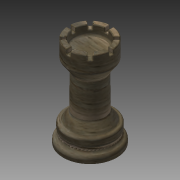
# Autodesk Inventor part: Castle
Saved by Autodesk Inventor 2015 SP1 (Build 190203100, 203)
## iProperties
Created: 2015-06-07
Part Number: Castle
Material: Generic
Document SubType Name: Modeling
Designer: Nathan
Density: 1 g/cm^3
Appearance: Driftwood
Author: Nathan
Autodesk Inventor part; units mm, degrees
ref_plane "YZ Plane" through (0, 0, 0) normal (1, 0, 0) x (0, 1, 0)
ref_plane "XZ Plane" through (0, 0, 0) normal (0, 1, 0) x (-1, 0, 0)
ref_plane "XY Plane" through (0, 0, 0) normal (0, 0, 1) x (1, 0, 0)
sketch "Sketch1" plane through (0, 0, 0) normal (0, 0, 1) x (1, 0, 0)
  line L0 (0, 47) -> (0, 0)
  line L1 (0, 0) -> (14.846, 0)
  arc A0 (12.9584, 6.4952) -> (13.7958, 3.4613) centre (14.831, 5.3796) ccw
  line L2 (13.2402, 9.7167) -> (13.2402, 7.5188)
  line L3 (14.846, 1.7013) -> (14.846, 0)
  arc A1 (12.9584, 6.4952) -> (13.2402, 7.5188) centre (11.2402, 7.5188) ccw
  arc A2 (14.846, 1.7013) -> (13.7958, 3.4613) centre (12.846, 1.7013) ccw
  arc A3 (13.2402, 9.7167) -> (12.1426, 10.7119) centre (12.2402, 9.7167) ccw
  arc A4 (11.2263, 11.133) -> (12.1426, 10.7119) centre (12.045, 11.7072) ccw
  line L4 (0, 0) -> (0, 50)
  line L5 (0, 50) -> (12.0578, 50)
  line L6 (12.0578, 50) -> (12.0578, 41.4087)
  line L7 (11.6943, 40.259) -> (8.3296, 35.4699)
  line L8 (7.9662, 34.2984) -> (8.1644, 16.1086)
  line L9 (8.5268, 14.982) -> (11.2263, 11.133)
  arc A5 (11.6943, 40.259) -> (12.0578, 41.4087) centre (10.0578, 41.4087) ccw
  arc A6 (8.3296, 35.4699) -> (7.9662, 34.2984) centre (9.9661, 34.3202) ccw
  arc A7 (8.1644, 16.1086) -> (8.5268, 14.982) centre (10.1642, 16.1304) ccw
  point P0 (14.846, 3.1999)
  point P1 (13.2402, 6.8697)
  point P2 (12.2402, 10.7167)
  point P3 (7.9592, 34.9427)
  point P4 (8.1711, 15.4891)
  dimension "d11" = 2
  dimension "d13" = 1
  dimension "d14" = 1
  dimension "d17" = 50
  dimension "d20" = 2
  constraints: 20 end point, 19 point on circle, 13 tangent, 8 centre point, 7 point on line, 3 equal radius, 2 horizontal, 2 vertical, 1 perpendicular
  measures "d11" radius of A1
  measures "d13" radius of A3
  measures "d14" radius of A4
  measures "d17" distance of L0.end L4.end
  measures "d20" radius of A5
revolve "Revolution1" add sketch "Sketch1" angle 360 about axis through (0, 47, 0) along (0, -1, 0)
sketch "Sketch2" plane through (0, 50, 0) normal (0, 1, 0) x (1, 0, 0)
  circle A0 centre (0, 0) radius 9
  dimension "d21" = 18
  constraints: 1 centre point, 1 coincident
  measures "d21" diameter of A0
extrude "Extrusion1" cut sketch "Sketch2" against normal blind 5
sketch "Sketch3" plane through (0, 50, 0) normal (0, 1, 0) x (1, 0, 0)
  line L0 (-1, -2.4142) -> (-12.1516, -13.5658)
  line L1 (-1, -18.185) -> (-1, -2.4142)
  line L2 (-2.4142, -1) -> (-18.185, -1)
  line L3 (-13.5658, -12.1516) -> (-2.4142, -1)
  line L4 (-2.4142, 1) -> (-13.5658, 12.1516)
  line L5 (-18.185, 1) -> (-2.4142, 1)
  line L6 (-1, 2.4142) -> (-1, 18.185)
  line L7 (-12.1516, 13.5658) -> (-1, 2.4142)
  line L8 (1, 2.4142) -> (12.1516, 13.5658)
  line L9 (1, 18.185) -> (1, 2.4142)
  line L10 (2.4142, 1) -> (18.185, 1)
  line L11 (13.5658, 12.1516) -> (2.4142, 1)
  line L12 (2.4142, -1) -> (13.5658, -12.1516)
  line L13 (18.185, -1) -> (2.4142, -1)
  line L14 (1, -2.4142) -> (1, -18.185)
  line L15 (12.1516, -13.5658) -> (1, -2.4142)
  arc A0 (-18.185, 1) -> (-18.185, -1) centre (0, 0) ccw
  arc A1 (-12.1516, 13.5658) -> (-13.5658, 12.1516) centre (0, 0) ccw
  arc A2 (1, 18.185) -> (-1, 18.185) centre (0, 0) ccw
  arc A3 (13.5658, 12.1516) -> (12.1516, 13.5658) centre (0, 0) ccw
  arc A4 (18.185, -1) -> (18.185, 1) centre (0, 0) ccw
  arc A5 (12.1516, -13.5658) -> (13.5658, -12.1516) centre (0, 0) ccw
  arc A6 (-13.5658, -12.1516) -> (-12.1516, -13.5658) centre (0, 0) ccw
  arc A7 (-1, -18.185) -> (1, -18.185) centre (0, 0) ccw
  dimension "d28" = 360
  constraints: 32 end point, 16 point on circle, 8 centre point
extrude "Extrusion2" cut sketch "Sketch3" against normal blind 2.5
fillet "Fillet1" radius 1 1 edges at (-9, 45, 0)
fillet "Fillet2" radius 0.5 98 edges at (-8.3149, 50, 3.4442) (-8.3149, 50, -3.4442) (-7.0317, 48.75, 5.6174) (-6.364, 47.5, 6.364) (-5.6174, 48.75, 7.0317) (-3.4442, 50, 8.3149) (-1, 48.75, 8.9443) (0, 47.5, 9) (1, 48.75, 8.9443) (3.4442, 50, 8.3149) (5.6174, 48.75, 7.0317) (6.364, 47.5, 6.364) (7.0317, 48.75, 5.6174) (8.3149, 50, 3.4442) (8.9443, 48.75, 1) (8.9861, 47.5, 0.5008) (8.9861, 47.5, -0.5008) (8.9443, 48.75, -1) (8.3149, 50, -3.4442) (7.0317, 48.75, -5.6174) (6.364, 47.5, -6.364) (5.6174, 48.75, -7.0317) (3.4442, 50, -8.3149) (1, 48.75, -8.9443) (0, 47.5, -9) (-1, 48.75, -8.9443) (-3.4442, 50, -8.3149) (-5.6174, 48.75, -7.0317) (-6.364, 47.5, -6.364) (-7.0317, 48.75, -5.6174) (-8.9443, 48.75, -1) (-9, 47.5, 0) (-8.9443, 48.75, 1) (-8.1178, 50, 6.7036) (-10.4803, 50, 1) (-11.14, 50, 4.6143) (-8.1178, 50, -6.7036) (-11.14, 50, -4.6143) (-10.4803, 50, -1) (-1, 50, -10.4803) (-4.6143, 50, -11.14) (-6.7036, 50, -8.1178) (6.7036, 50, -8.1178) (4.6143, 50, -11.14) (1, 50, -10.4803) (10.4803, 50, -1) (11.14, 50, -4.6143) (8.1178, 50, -6.7036) (-9.2039, 48.75, 7.7897) (-12.0163, 48.75, 1) (-12.0578, 47.5, 0) (-12.0163, 48.75, -1) (-9.2039, 48.75, -7.7897) (-8.5261, 47.5, -8.5261) (-7.7897, 48.75, -9.2039) (-1, 48.75, -12.0163) (0, 47.5, -12.0578) (1, 48.75, -12.0163) (7.7897, 48.75, -9.2039) (8.5261, 47.5, -8.5261) (9.2039, 48.75, -7.7897) (12.0163, 48.75, -1) (12.0474, 47.5, -0.5004) (12.0474, 47.5, 0.5004) (12.0163, 48.75, 1) (11.14, 50, 4.6143) (9.2039, 48.75, 7.7897) (8.5261, 47.5, 8.5261) (7.7897, 48.75, 9.2039) (4.6143, 50, 11.14) (1, 48.75, 12.0163) (0, 47.5, 12.0578) (-1, 48.75, 12.0163) (-4.6143, 50, 11.14) (-7.7897, 48.75, 9.2039) (-8.5261, 47.5, 8.5261) (8.1178, 50, 6.7036) (10.4803, 50, 1) (1, 50, 10.4803) (6.7036, 50, 8.1178) (-1, 47.5, 10.4803) (-1, 50, 10.4803) (-6.7036, 50, 8.1178) (-8.1178, 47.5, 6.7036) (-6.7036, 47.5, 8.1178) (1, 47.5, 10.4803) (10.4803, 47.5, -1) (10.4803, 47.5, 1) (6.7036, 47.5, -8.1178) (8.1178, 47.5, -6.7036) (-1, 47.5, -10.4803) (1, 47.5, -10.4803) (-8.1178, 47.5, -6.7036) (-6.7036, 47.5, -8.1178) (-10.4803, 47.5, 1) (-10.4803, 47.5, -1) (8.1178, 47.5, 6.7036) (6.7036, 47.5, 8.1178)
body "Solid1"
